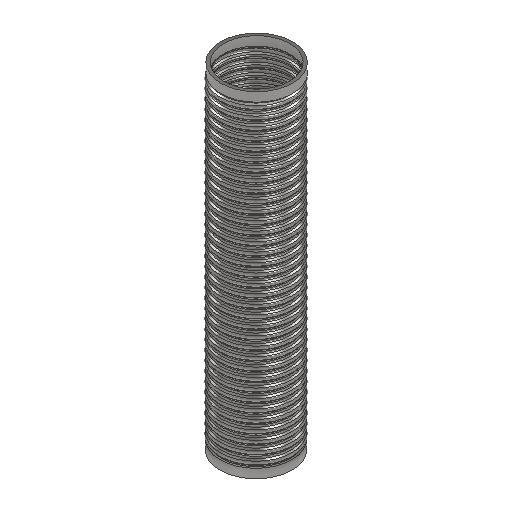
# Autodesk Inventor part: bellows_bellows
Saved by Autodesk Inventor 2026.3 (Build 303398000, 398)
## iProperties
Created: 2026-05-14
Part Number: bellows_bellows
Material: ステンレス鋼 440C
Document SubType Name: Modeling
Designer: shusu
Density: 7.75 g/cm^3
Appearance: 半つや出し
Author: shusu
Autodesk Inventor part; units mm, degrees
ref_plane "YZ Plane" through (0, 0, 0) normal (1, 0, 0) x (0, 1, 0)
ref_plane "XZ Plane" through (0, 0, 0) normal (0, 1, 0) x (-1, 0, 0)
ref_plane "XY Plane" through (0, 0, 0) normal (0, 0, 1) x (1, 0, 0)
sketch "スケッチ1" plane through (0, 0, 0) normal (0, 1, 0) x (-1, 0, 0)
  circle A0 centre (0, 0) radius 30
  dimension "d0" = 60
  constraints: 1 centre point, 1 coincident
  measures "d0" diameter of A0
sketch "スケッチ2" plane through (0, 0, 0) normal (1, 0, 0) x (0, 1, 0)
  line L0 (0, -29.172) -> (0, -30.0004)
  line L1 (2.5858, -31.7578) -> (1.4142, -30.5862)
  line L2 (0, -29.172) -> (0, -29.0004)
  line L3 (1.4142, -29.5862) -> (2.5858, -30.7578)
  line L4 (5.4142, -31.7578) -> (6.586, -30.586)
  line L5 (6.586, -29.586) -> (5.4142, -30.7578)
  arc A0 (8, -29.0002) -> (6.586, -29.586) centre (8.0002, -31.0002) ccw
  arc A1 (8, -30.0002) -> (6.586, -30.586) centre (8.0002, -32.0002) ccw
  arc A2 (2.5858, -30.7578) -> (5.4142, -30.7578) centre (4, -29.3436) ccw
  arc A3 (2.5858, -31.7578) -> (5.4142, -31.7578) centre (4, -30.3436) ccw
  arc A4 (1.4142, -29.5862) -> (0, -29.0004) centre (0, -31.0004) ccw
  arc A5 (1.4142, -30.5862) -> (0, -30.0004) centre (0, -32.0004) ccw
  line L6 (8, -30.0002) -> (8, -29.0002)
  point P0 (0, 0)
  point P1 (-4, -22.172)
  point P2 (8, -28.172)
  point P3 (12, -22.172)
  constraints: 14 end point, 12 point on circle, 8 tangent, 6 centre point, 5 equal radius, 2 point on line, 1 vertical
sweep "スイープ1" add profiles "スケッチ2" path "スケッチ1"
pattern_linear "矩形状パターン1" count 35 spacing 8 along (0, 1, 0) of "スイープ1"
sketch "スケッチ8" plane through (0, 0, 0) normal (0, -1, 0) x (1, 0, 0)
  point P0 (0, 0)
sketch "スケッチ9" plane through (0, 0, 0) normal (0, -1, 0) x (1, 0, 0)
  circle A0 centre (0, 0) radius 29.0004
  circle A1 centre (0, 0) radius 31.75
  dimension "d25" = 63.5
  constraints: 2 centre point, 2 coincident
  measures "d25" diameter of A1
extrude "押し出し6" add sketch "スケッチ9" along normal blind 8
sketch "スケッチ11" plane through (0, 280, 0) normal (0, 1, 0) x (1, 0, 0)
  circle A0 centre (0.2054, 0.3798) radius 29.0004
  circle A1 centre (0.2054, 0.3798) radius 31.75
  point P0 (0, 0)
  dimension "d31" = 63.5
  constraints: 2 centre point, 2 coincident
  measures "d31" diameter of A1
extrude "押し出し8" add sketch "スケッチ11" along normal blind 8
